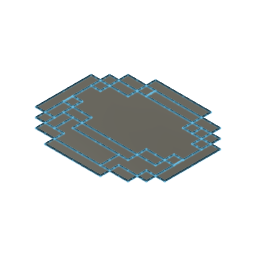
Compass_Body (Autodesk Fusion 360 archive; units mm, degrees)
design "Compass_Top"
Autodesk Fusion 360 part; units mm, degrees
sketch "Sketch1" plane through (0, 0, 0) normal (0, 0, 1) x (1, 0, 0)
  line L0 (111.033, 142.8577) -> (81.033, 142.8577)
  line L1 (81.033, 137.8577) -> (81.033, 132.8577)
  line L2 (91.033, 137.8577) -> (91.033, 132.8577)
  line L3 (81.033, 132.8577) -> (81.033, 137.8577)
  line L4 (81.033, 42.8579) -> (111.033, 42.8579)
  line L5 (111.033, 32.858) -> (81.033, 32.858)
  line L6 (81.033, 72.8579) -> (111.033, 72.8579)
  line L7 (111.033, 72.8579) -> (81.033, 72.8579)
  line L8 (91.033, 142.8577) -> (116.0329, 142.8577)
  line L9 (106.033, 42.8579) -> (81.033, 42.8579)
  line L10 (61.0331, 132.8577) -> (61.0331, 137.8577)
  line L11 (141.0329, 137.8577) -> (141.0329, 132.8577)
  line L12 (91.033, 132.8577) -> (91.033, 137.8577)
  line L13 (161.0329, 137.8577) -> (161.0329, 132.8577)
  line L14 (51.0331, 122.8578) -> (56.0331, 122.8578)
  line L15 (56.0331, 62.8579) -> (51.0331, 62.8579)
  line L16 (161.0329, 117.8578) -> (161.0329, 112.8578)
  line L17 (161.0329, 47.858) -> (161.0329, 42.8579)
  line L18 (161.0329, 42.8579) -> (151.0329, 42.8579)
  line L19 (171.0328, 87.8578) -> (171.0328, 82.8579)
  line L20 (161.0329, 82.8579) -> (161.0329, 87.8578)
  line L21 (141.0329, 47.8579) -> (141.0329, 52.8579)
  line L22 (171.0328, 92.8578) -> (171.0328, 87.8578)
  line L23 (61.0331, 77.8579) -> (61.0331, 82.8579)
  line L24 (141.0329, 52.8579) -> (141.0329, 47.8579)
  line L25 (141.0329, 37.858) -> (141.0329, 32.858)
  line L26 (141.0329, 67.8579) -> (141.0329, 62.8579)
  line L27 (161.0329, 82.8579) -> (166.0328, 82.8579)
  line L28 (81.033, 72.8579) -> (81.033, 77.8579)
  line L29 (171.0328, 57.8579) -> (171.0328, 52.858)
  line L30 (151.0329, 82.8579) -> (161.0329, 82.8579)
  line L31 (161.0329, 77.8579) -> (161.0329, 72.8579)
  line L32 (161.0329, 82.8579) -> (161.0329, 77.8579)
  line L33 (161.0329, 87.8578) -> (161.0329, 92.8578)
  line L34 (166.0328, 52.858) -> (161.0329, 52.8579)
  line L35 (161.0329, 112.8578) -> (161.0329, 117.8578)
  line L36 (71.033, 72.8579) -> (76.0331, 72.8579)
  line L37 (146.0329, 122.8578) -> (141.0329, 122.8578)
  line L38 (61.0331, 57.8579) -> (61.0331, 52.858)
  line L39 (161.0329, 122.8578) -> (166.0328, 122.8578)
  line L40 (176.0328, 62.8579) -> (171.0328, 62.8579)
  line L41 (171.0328, 102.8578) -> (171.0328, 92.8578)
  line L42 (166.0328, 122.8578) -> (161.0329, 122.8578)
  line L43 (61.0331, 92.8578) -> (56.0331, 92.8578)
  line L44 (171.0328, 52.858) -> (166.0328, 52.858)
  line L45 (81.033, 52.858) -> (76.0331, 52.858)
  line L46 (81.033, 77.8579) -> (81.033, 72.8579)
  line L47 (141.0329, 77.8579) -> (141.0329, 82.8579)
  line L48 (71.033, 82.8579) -> (81.033, 82.8579)
  line L49 (61.0331, 52.858) -> (71.033, 52.858)
  line L50 (141.0329, 72.8579) -> (141.0329, 77.8579)
  line L51 (141.0329, 72.8579) -> (151.0329, 72.8579)
  line L52 (61.0331, 92.8578) -> (61.0331, 87.8578)
  line L53 (141.0329, 82.8579) -> (141.0329, 77.8579)
  line L54 (166.0328, 92.8578) -> (161.0329, 92.8578)
  line L55 (61.0331, 82.8579) -> (61.0331, 72.8579)
  line L56 (61.0331, 132.8577) -> (61.0331, 127.8577)
  line L57 (71.033, 52.858) -> (81.033, 52.858)
  line L58 (136.0329, 62.8579) -> (141.0329, 62.8579)
  line L59 (61.0331, 82.8579) -> (71.033, 82.8579)
  line L60 (66.0331, 72.8579) -> (71.033, 72.8579)
  line L61 (161.0329, 132.8577) -> (166.0328, 132.8577)
  line L62 (71.033, 52.858) -> (66.0331, 52.858)
  line L63 (161.0329, 112.8578) -> (166.0328, 112.8578)
  line L64 (161.0329, 72.8579) -> (161.0329, 77.8579)
  line L65 (61.0331, 72.8579) -> (61.0331, 77.8579)
  line L66 (151.0329, 42.8579) -> (141.0329, 42.8579)
  line L67 (141.0329, 77.8579) -> (141.0329, 72.8579)
  line L68 (171.0328, 62.8579) -> (166.0328, 62.8579)
  line L69 (141.0329, 52.8579) -> (151.0329, 52.8579)
  line L70 (161.0329, 62.8579) -> (161.0329, 57.8579)
  line L71 (181.0328, 62.8579) -> (176.0328, 62.8579)
  line L72 (161.0329, 132.8577) -> (161.0329, 127.8578)
  line L73 (166.0328, 122.8578) -> (171.0328, 122.8578)
  line L74 (71.033, 62.8579) -> (71.033, 52.858)
  line L75 (56.0331, 62.8579) -> (61.0331, 62.8579)
  line L76 (171.0328, 92.8578) -> (166.0328, 92.8578)
  line L77 (151.0329, 52.8579) -> (161.0329, 52.8579)
  line L78 (161.0329, 62.8579) -> (166.0328, 62.8579)
  line L79 (161.0329, 52.8579) -> (151.0329, 52.8579)
  line L80 (171.0328, 82.8579) -> (166.0328, 82.8579)
  line L81 (81.033, 42.8579) -> (71.033, 42.8579)
  line L82 (81.033, 72.8579) -> (81.033, 67.8579)
  line L83 (56.0331, 82.8579) -> (61.0331, 82.8579)
  line L84 (161.0329, 127.8578) -> (161.0329, 132.8577)
  line L85 (71.033, 82.8579) -> (61.0331, 82.8579)
  line L86 (61.0331, 47.858) -> (61.0331, 52.858)
  line L87 (51.0331, 57.8579) -> (51.0331, 62.8579)
  line L88 (41.0331, 122.8578) -> (46.0331, 122.8578)
  line L89 (61.0331, 52.858) -> (56.0331, 52.858)
  line L90 (61.0331, 132.8577) -> (71.033, 132.8577)
  line L91 (141.0329, 42.8579) -> (136.0329, 42.8579)
  line L92 (151.0329, 72.8579) -> (161.0329, 72.8579)
  line L93 (41.0331, 62.8579) -> (41.0331, 92.8578)
  line L94 (81.033, 132.8577) -> (81.033, 127.8577)
  line L95 (171.0328, 82.8579) -> (171.0328, 72.8579)
  line L96 (81.033, 47.858) -> (81.033, 52.858)
  line L97 (81.033, 42.8579) -> (81.033, 47.858)
  line L98 (166.0328, 132.8577) -> (171.0328, 132.8577)
  line L99 (141.0329, 42.8579) -> (141.0329, 37.858)
  line L100 (61.0331, 87.8578) -> (61.0331, 82.8579)
  line L101 (51.0331, 82.8579) -> (51.0331, 87.8578)
  line L102 (151.0329, 127.8578) -> (151.0329, 122.8578)
  line L103 (141.0329, 62.8579) -> (141.0329, 67.8579)
  line L104 (51.0331, 92.8578) -> (51.0331, 102.8578)
  line L105 (151.0329, 132.8577) -> (151.0329, 127.8578)
  line L106 (141.0329, 127.8578) -> (141.0329, 132.8577)
  line L107 (161.0329, 52.8579) -> (161.0329, 47.858)
  line L108 (151.0329, 122.8578) -> (146.0329, 122.8578)
  line L109 (71.033, 72.8579) -> (61.0331, 72.8579)
  line L110 (171.0328, 127.8578) -> (171.0328, 122.8578)
  line L111 (161.0329, 122.8578) -> (161.0329, 127.8578)
  line L112 (61.0331, 122.8578) -> (71.033, 122.8578)
  line L113 (176.0328, 122.8578) -> (181.0328, 122.8578)
  line L114 (161.0329, 82.8579) -> (151.0329, 82.8579)
  line L115 (81.033, 37.858) -> (81.033, 42.8579)
  line L116 (61.0331, 62.8579) -> (61.0331, 57.8579)
  line L117 (56.0331, 112.8578) -> (61.0331, 112.8578)
  line L118 (146.0329, 132.8577) -> (151.0329, 132.8577)
  line L119 (161.0329, 57.8579) -> (161.0329, 52.8579)
  line L120 (161.0329, 122.8578) -> (161.0329, 117.8578)
  line L121 (81.033, 82.8579) -> (81.033, 77.8579)
  line L122 (171.0328, 62.8579) -> (171.0328, 57.8579)
  line L123 (76.0331, 72.8579) -> (81.033, 72.8579)
  line L124 (161.0329, 92.8578) -> (161.0329, 87.8578)
  line L125 (151.0329, 132.8577) -> (141.0329, 132.8577)
  line L126 (151.0329, 82.8579) -> (141.0329, 82.8579)
  line L127 (76.0331, 52.858) -> (71.033, 52.858)
  line L128 (81.033, 127.8577) -> (81.033, 132.8577)
  line L129 (81.033, 67.8579) -> (81.033, 72.8579)
  line L130 (51.0331, 62.8579) -> (46.0331, 62.8579)
  line L131 (56.0331, 122.8578) -> (61.0331, 122.8578)
  line L132 (161.0329, 92.8578) -> (166.0328, 92.8578)
  line L133 (61.0331, 117.8578) -> (61.0331, 112.8578)
  line L134 (81.033, 82.8579) -> (71.033, 82.8579)
  line L135 (81.033, 122.8578) -> (81.033, 127.8577)
  line L136 (61.0331, 122.8578) -> (61.0331, 117.8578)
  line L137 (81.033, 72.8579) -> (71.033, 72.8579)
  line L138 (151.0329, 122.8578) -> (151.0329, 127.8578)
  line L139 (81.033, 122.8578) -> (71.033, 122.8578)
  line L140 (51.0331, 62.8579) -> (51.0331, 72.8579)
  line L141 (81.033, 47.858) -> (81.033, 42.8579)
  line L142 (81.033, 152.8577) -> (111.033, 152.8577)
  line L143 (141.0329, 132.8577) -> (141.0329, 127.8578)
  line L144 (141.0329, 82.8579) -> (151.0329, 82.8579)
  line L145 (91.033, 132.8577) -> (86.033, 132.8577)
  line L146 (171.0328, 112.8578) -> (166.0328, 112.8578)
  line L147 (151.0329, 72.8579) -> (141.0329, 72.8579)
  line L148 (81.033, 127.8577) -> (81.033, 122.8578)
  line L149 (61.0331, 87.8578) -> (61.0331, 92.8578)
  line L150 (161.0329, 57.8579) -> (161.0329, 62.8579)
  line L151 (71.033, 52.858) -> (71.033, 62.8579)
  line L152 (171.0328, 117.8578) -> (171.0328, 112.8578)
  line L153 (166.0328, 112.8578) -> (161.0329, 112.8578)
  line L154 (161.0329, 72.8579) -> (151.0329, 72.8579)
  line L155 (141.0329, 122.8578) -> (141.0329, 127.8578)
  line L156 (71.033, 42.8579) -> (61.0331, 42.8579)
  line L157 (161.0329, 87.8578) -> (161.0329, 82.8579)
  line L158 (81.033, 52.858) -> (81.033, 47.858)
  line L159 (161.0329, 127.8578) -> (161.0329, 122.8578)
  line L160 (166.0328, 112.8578) -> (171.0328, 112.8578)
  line L161 (151.0329, 52.8579) -> (141.0329, 52.8579)
  line L162 (161.0329, 117.8578) -> (161.0329, 122.8578)
  line L163 (151.0329, 127.8578) -> (151.0329, 132.8577)
  line L164 (81.033, 77.8579) -> (81.033, 82.8579)
  line L165 (61.0331, 62.8579) -> (56.0331, 62.8579)
  line L166 (166.0328, 62.8579) -> (161.0329, 62.8579)
  line L167 (61.0331, 72.8579) -> (66.0331, 72.8579)
  line L168 (171.0328, 122.8578) -> (176.0328, 122.8578)
  line L169 (56.0331, 92.8578) -> (61.0331, 92.8578)
  line L170 (141.0329, 132.8577) -> (146.0329, 132.8577)
  line L171 (61.0331, 82.8579) -> (61.0331, 87.8578)
  line L172 (86.033, 132.8577) -> (81.033, 132.8577)
  line L173 (66.0331, 52.858) -> (61.0331, 52.858)
  line L174 (61.0331, 122.8578) -> (56.0331, 122.8578)
  line L175 (161.0329, 52.8579) -> (161.0329, 57.8579)
  line L176 (166.0328, 82.8579) -> (171.0328, 82.8579)
  line L177 (141.0329, 47.8579) -> (141.0329, 42.8579)
  line L178 (156.0329, 122.8578) -> (151.0329, 122.8578)
  line L179 (171.0328, 132.8577) -> (171.0328, 127.8578)
  line L180 (171.0328, 122.8578) -> (171.0328, 117.8578)
  line L181 (141.0329, 42.8579) -> (141.0329, 47.8579)
  line L182 (61.0331, 112.8578) -> (61.0331, 117.8578)
  line L183 (141.0329, 122.8578) -> (151.0329, 122.8578)
  line L184 (166.0328, 82.8579) -> (161.0329, 82.8579)
  line L185 (61.0331, 127.8577) -> (61.0331, 132.8577)
  line L186 (61.0331, 42.8579) -> (61.0331, 47.858)
  line L187 (151.0329, 132.8577) -> (156.0329, 132.8577)
  line L188 (81.033, 32.858) -> (81.033, 37.858)
  line L189 (71.033, 132.8577) -> (61.0331, 132.8577)
  line L190 (161.0329, 77.8579) -> (161.0329, 82.8579)
  line L191 (61.0331, 52.858) -> (61.0331, 62.8579)
  line L192 (141.0329, 127.8578) -> (141.0329, 122.8578)
  line L193 (166.0328, 62.8579) -> (171.0328, 62.8579)
  line L194 (61.0331, 127.8577) -> (61.0331, 122.8578)
  line L195 (61.0331, 82.8579) -> (56.0331, 82.8579)
  line L196 (171.0328, 122.8578) -> (166.0328, 122.8578)
  line L197 (166.0328, 92.8578) -> (171.0328, 92.8578)
  line L198 (81.033, 132.8577) -> (111.033, 132.8577)
  line L199 (116.0329, 132.8577) -> (91.033, 132.8577)
  line L200 (111.033, 62.8579) -> (81.033, 62.8579)
  line L201 (81.033, 62.8579) -> (106.033, 62.8579)
  line L202 (131.0329, 52.858) -> (131.0329, 42.8579)
  line L203 (131.0329, 52.858) -> (131.0329, 62.8579)
  line L204 (91.033, 137.8577) -> (91.033, 142.8577)
  line L205 (41.0331, 92.8578) -> (41.0331, 122.8578)
  line L206 (131.0329, 42.8579) -> (106.033, 42.8579)
  line L207 (51.0331, 102.8578) -> (51.0331, 112.8578)
  line L208 (161.0329, 142.8577) -> (161.0329, 137.8577)
  line L209 (51.0331, 92.8578) -> (51.0331, 62.8579)
  line L210 (141.0329, 137.8577) -> (141.0329, 142.8577)
  line L211 (51.0331, 122.8578) -> (51.0331, 92.8578)
  line L212 (61.0331, 72.8579) -> (61.0331, 62.8579)
  line L213 (46.0331, 122.8578) -> (51.0331, 122.8578)
  line L214 (181.0328, 92.8578) -> (181.0328, 62.8579)
  line L215 (141.0329, 142.8577) -> (141.0329, 137.8577)
  line L216 (56.0331, 132.8577) -> (61.0331, 132.8577)
  line L217 (181.0328, 122.8578) -> (181.0328, 92.8578)
  line L218 (141.0329, 67.8579) -> (141.0329, 72.8579)
  line L219 (156.0329, 132.8577) -> (161.0329, 132.8577)
  line L220 (61.0331, 122.8578) -> (61.0331, 127.8577)
  line L221 (141.0329, 152.8577) -> (141.0329, 147.8577)
  line L222 (131.0329, 62.8579) -> (131.0329, 52.858)
  line L223 (171.0328, 92.8578) -> (171.0328, 122.8578)
  line L224 (81.033, 147.8577) -> (81.033, 152.8577)
  line L225 (151.0329, 142.8577) -> (161.0329, 142.8577)
  line L226 (141.0329, 147.8577) -> (141.0329, 142.8577)
  line L227 (171.0328, 72.8579) -> (171.0328, 62.8579)
  line L228 (71.033, 132.8577) -> (81.033, 132.8577)
  line L229 (51.0331, 112.8578) -> (51.0331, 117.8578)
  line L230 (151.0329, 122.8578) -> (161.0329, 122.8578)
  line L231 (71.033, 62.8579) -> (71.033, 72.8579)
  line L232 (171.0328, 112.8578) -> (171.0328, 102.8578)
  line L233 (71.033, 122.8578) -> (81.033, 122.8578)
  line L234 (46.0331, 62.8579) -> (41.0331, 62.8579)
  line L235 (106.033, 62.8579) -> (131.0329, 62.8579)
  line L236 (71.033, 122.8578) -> (61.0331, 122.8578)
  line L237 (131.0329, 42.8579) -> (131.0329, 52.858)
  line L238 (61.0331, 62.8579) -> (61.0331, 72.8579)
  line L239 (61.0331, 112.8578) -> (56.0331, 112.8578)
  line L240 (161.0329, 132.8577) -> (151.0329, 132.8577)
  line L241 (71.033, 72.8579) -> (71.033, 62.8579)
  line L242 (51.0331, 127.8578) -> (51.0331, 132.8577)
  line L243 (81.033, 62.8579) -> (81.033, 67.8579)
  line L244 (51.0331, 117.8578) -> (51.0331, 122.8578)
  line L245 (161.0329, 122.8578) -> (156.0329, 122.8578)
  line L246 (51.0331, 87.8578) -> (51.0331, 92.8578)
  line L247 (51.0331, 72.8579) -> (51.0331, 82.8579)
  line L248 (141.0329, 72.8579) -> (141.0329, 67.8579)
  line L249 (61.0331, 117.8578) -> (61.0331, 122.8578)
  line L250 (81.033, 67.8579) -> (81.033, 62.8579)
  line L251 (51.0331, 122.8578) -> (51.0331, 127.8578)
  line L252 (81.033, 132.8577) -> (71.033, 132.8577)
  line L253 (51.0331, 52.858) -> (51.0331, 57.8579)
  line L254 (171.0328, 62.8579) -> (171.0328, 92.8578)
  line L255 (141.0329, 72.8579) -> (111.033, 72.8579)
  line L256 (51.0331, 62.8579) -> (56.0331, 62.8579)
  line L257 (111.033, 72.8579) -> (141.0329, 72.8579)
  line L258 (81.033, 142.8577) -> (86.033, 142.8577)
  line L259 (141.0329, 142.8577) -> (111.033, 142.8577)
  line L260 (141.0329, 132.8577) -> (141.0329, 137.8577)
  line L261 (51.0331, 92.8578) -> (56.0331, 92.8578)
  line L262 (51.0331, 112.8578) -> (56.0331, 112.8578)
  line L263 (61.0331, 142.8577) -> (71.033, 142.8577)
  line L264 (61.0331, 137.8577) -> (61.0331, 142.8577)
  line L265 (56.0331, 122.8578) -> (51.0331, 122.8578)
  line L266 (81.033, 137.8577) -> (81.033, 142.8577)
  line L267 (86.033, 142.8577) -> (91.033, 142.8577)
  line L268 (56.0331, 112.8578) -> (51.0331, 112.8578)
  line L269 (111.033, 152.8577) -> (141.0329, 152.8577)
  line L270 (141.0329, 32.858) -> (111.033, 32.858)
  line L271 (116.0329, 142.8577) -> (141.0329, 142.8577)
  line L272 (56.0331, 92.8578) -> (51.0331, 92.8578)
  line L273 (131.0329, 62.8579) -> (136.0329, 62.8579)
  line L274 (136.0329, 42.8579) -> (131.0329, 42.8579)
  line L275 (111.033, 132.8577) -> (141.0329, 132.8577)
  line L276 (141.0329, 62.8579) -> (111.033, 62.8579)
  line L277 (91.033, 142.8577) -> (91.033, 137.8577)
  line L278 (81.033, 142.8577) -> (81.033, 147.8577)
  line L279 (81.033, 142.8577) -> (81.033, 137.8577)
  line L280 (141.0329, 142.8577) -> (151.0329, 142.8577)
  line L281 (51.0331, 82.8579) -> (56.0331, 82.8579)
  line L282 (111.033, 42.8579) -> (141.0329, 42.8579)
  line L283 (56.0331, 52.858) -> (51.0331, 52.858)
  line L284 (141.0329, 132.8577) -> (116.0329, 132.8577)
  line L285 (56.0331, 82.8579) -> (51.0331, 82.8579)
  line L286 (51.0331, 132.8577) -> (56.0331, 132.8577)
  line L287 (71.033, 142.8577) -> (81.033, 142.8577)
extrude "Extrude1" add sketch "Sketch1" along normal blind 0.4 contours L6 L7 L16 L20 L28 L30 L33 L35 L37 L41 L43 L46 L47 L48 L50 L52 L53 L54 L59 L63 L67 L76 L85 L94 L100 L104 L106 L108 L112 L114 L117 L120 L121 L124 L126 L128 L132 L133 L134 L135 L136 L139 L143 L144 L145 L146 L148 L149 L153 L155 L157 L160 L162 L164 L169 L171 L172 L178 L182 L183 L192 L197 L198 L199 L207 L211 L223 L230 L232 L233 L236 L239 L245 L249 L255 L257 L261 L262 L268 L272 L275 L284 | L21 L24 L26 L27 L31 L32 L51 L58 L64 L68 L69 L70 L77 L78 L79 L80 L91 L92 L95 L103 L119 L147 L150 L154 L161 L166 L175 L176 L177 L181 L184 L190 L193 L202 L203 L218 L222 L227 L237 L248 L254 L273 L274 L276 L282 makes body 1 in component "Component"
extrude "Extrude1'" add sketch "Sketch1" along normal blind 0.4 separate body contours L0 L8 L142 L221 L224 L226 L258 L259 L267 L269 L271 L278 | L11 L13 L118 L125 L170 L187 L208 L210 L215 L219 L225 L240 L260 L280 | L1 L3 L10 L90 L189 L228 L252 L263 L264 L266 L279 L287 | L39 L42 L61 L72 L73 L84 L98 L110 L111 L159 L179 L196 | L14 L56 L131 L174 L185 L194 L216 L220 L242 L251 L265 L286 | L19 L22 L40 L41 L71 L95 L113 L152 L168 L180 L214 L217 L223 L227 L232 L254 | L88 L93 L101 L104 L130 L140 L205 L207 L209 L211 L213 L229 L234 L244 L246 L247 | L19 L20 L22 L27 L33 L54 L76 L80 L124 L132 L157 L176 L184 L197 L254 | L43 L52 L83 L100 L101 L149 L169 L171 L195 L209 L246 L261 L272 L281 L285 | L29 L34 L44 L68 L70 L78 L119 L122 L150 L166 L175 L193 | L15 L38 L75 L87 L89 L116 L165 L191 L253 L256 L283 | L30 L31 L32 L47 L50 L51 L53 L64 L67 L92 L114 L126 L144 L147 L154 L190 | L23 L28 L36 L46 L48 L55 L59 L60 L65 L85 L109 L121 L123 L134 L137 L164 L167 | L17 L18 L21 L24 L66 L69 L77 L79 L107 L161 L177 L181 | L45 L49 L57 L62 L81 L86 L96 L97 L127 L141 L156 L158 L173 L186 | L6 L7 L26 L58 L82 L103 L129 L200 L201 L218 L235 L243 L248 L250 L255 L257 L273 L276 | L4 L5 L9 L25 L91 L99 L115 L188 L206 L270 L274 L282 makes body 2 in component "Component'"
extrude "Extrude1''" add sketch "Sketch1" along normal blind 0.4 separate body contours L0 L2 L8 L11 L12 L198 L199 L204 L210 L215 L259 L260 L271 L275 L277 L284 | L0 L1 L2 L3 L12 L145 L172 L198 L204 L258 L266 L267 L277 L279 | L37 L102 L105 L106 L108 L118 L125 L138 L143 L155 L163 L170 L183 L192 | L56 L90 L94 L112 L128 L135 L139 L148 L185 L189 L194 L220 L228 L233 L236 L252 | L16 L35 L39 L42 L63 L73 L120 L146 L152 L153 L160 L162 L180 L196 L223 | L14 L117 L131 L133 L136 L174 L182 L211 L229 L239 L244 L249 L262 L265 L268 | L15 L23 L55 L65 L75 L83 L140 L165 L195 L209 L212 L238 L247 L256 L281 L285 | L4 L9 L36 L45 L57 L74 L82 L96 L97 L123 L127 L129 L137 L141 L151 L158 L200 L201 L202 L203 L206 L222 L231 L235 L237 L241 L243 L250 L276 L282 makes body 3 at (94.3663, 139.5244, 0) makes body 3 at (74.3664, 129.5244, 0) makes body 3 at (147.6995, 127.8578, 0) makes body 3 at (57.6997, 119.5244, 0) makes body 5 at (166.0328, 116.1911, 0) makes body 4 at (54.3664, 72.8579, 0) makes body 6 at (114.3663, 52.8579, 0) in component "Component''"
extrude "Extrude1'''" add sketch "Sketch1" along normal blind 0.4 separate body contours L72 L84 L102 L105 L111 L138 L159 L163 L178 L187 L219 L230 L240 L245 | L38 L49 L60 L62 L74 L109 L116 L151 L167 L173 L191 L212 L231 L238 L241 makes body 7 at (67.6997, 62.8579, 0) makes body 8 at (154.3662, 129.5244, 0) in component "Component'''"
component "Component" placed x (1, 0, 0) y (0, 1, 0) z (0, 0, 1) at (0, 0, 0)
component "Component'" placed x (1, 0, 0) y (0, 1, 0) z (0, 0, 1) at (0, 0, 0)
component "Component''" placed x (1, 0, 0) y (0, 1, 0) z (0, 0, 1) at (0, 0, 0)
component "Component'''" placed x (1, 0, 0) y (0, 1, 0) z (0, 0, 1) at (0, 0, 0)
